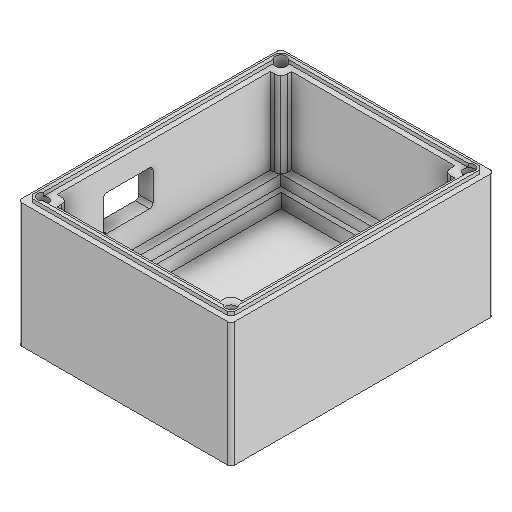
# Autodesk Inventor part: Box_bottom_v2
Saved by Autodesk Inventor 2026.1 (Build 301233020, 233B)
## iProperties
Created: 2025-09-17
Part Number: Box_bottom_v2
Material: Generic
Document SubType Name: Modeling
Designer: samuel
Density: 1 g/cm^3
Appearance: Default
Author: samuel
Autodesk Inventor part; units mm, degrees
ref_plane "YZ Plane" through (0, 0, 0) normal (1, 0, 0) x (0, 1, 0)
ref_plane "XZ Plane" through (0, 0, 0) normal (0, 1, 0) x (-1, 0, 0)
ref_plane "XY Plane" through (0, 0, 0) normal (0, 0, 1) x (1, 0, 0)
sketch "Sketch2" plane through (0, 0, 0) normal (0, 0, 1) x (1, 0, 0)
  line L0 (-30, -27) -> (30, -27)
  line L1 (30, -27) -> (30, 27)
  line L2 (30, 27) -> (-30, 27)
  line L3 (-30, 27) -> (-30, -27)
  line L4 (-30, -27) -> (30, 27) construction
  line L5 (30, -27) -> (-30, 27) construction
  line L6 (-30, 27) -> (30, 27)
  line L7 (30, 27) -> (30, 47)
  line L8 (30, 47) -> (-30, 47)
  line L9 (-30, 47) -> (-30, 27)
  line L10 (-25, -22) -> (25, -22)
  line L11 (25, -22) -> (25, 22)
  line L12 (25, 22) -> (-25, 22)
  line L13 (-25, 22) -> (-25, -22)
  point P0 (0, 0)
  dimension "d4" = 60
  dimension "d5" = 54
  dimension "d48" = 20
  dimension "d142" = 5
  constraints: 28 end point, 6 parallel, 3 perpendicular, 2 horizontal, 2 midpoint, 3 other
  measures "d4" distance of L2.end L1.end
  measures "d5" distance of L0.end L1.end
  measures "d48" distance of L7.end L6.end
  measures "d142" distance between parallel lines of L3 L13
extrude "Extrusion2" add sketch "Sketch2" along normal blind 35 contours L3 L2 L1 L0 | L9 L8 L7 L2 | L13 L12 L11 L10
shell "Shell1" thickness 4 removed faces 1 at (-10, 22.3333, 35)
sketch "Sketch11" plane through (-30, -27, 0) normal (-1, 0, 0) x (0, 0, 1)
  line L0 (28.5, 34) -> (18.5, 34)
  line L1 (18.5, 34) -> (18.5, 20)
  line L2 (18.5, 20) -> (28.5, 20)
  line L3 (28.5, 20) -> (28.5, 34)
  line L4 (28.5, 34) -> (18.5, 20) construction
  line L5 (18.5, 34) -> (28.5, 20) construction
  line L6 (0, 0) -> (35, 0) projected
  line L7 (0, 74) -> (0, 0) projected
  point P0 (0, 27)
  point P1 (23.5, 27)
  dimension "d65" = 10
  dimension "d66" = 14
  dimension "d67" = 20
  dimension "d68" = 18.5
  constraints: 12 end point, 2 midpoint, 2 parallel, 1 horizontal, 1 perpendicular
  measures "d65" distance of L2.end L1.end
  measures "d66" distance of L1.end L0.end
  measures "d67" distance between parallel lines of L6 L2
  measures "d68" distance between parallel lines of L7 L1
extrude "Extrusion9" cut sketch "Sketch11" against normal blind 5
sketch "Sketch12" plane through (-26, 43, 4) normal (0, 0, 1) x (1, 0, 0)
  line L0 (0, 0) -> (52, 0) projected
  line L1 (52, 0) -> (49, 0)
  line L2 (49, 0) -> (49, -3)
  line L3 (49, -3) -> (52, -3)
  line L4 (52, -3) -> (52, 0)
  line L5 (52, -66) -> (52, 0) projected
  line L6 (52, -66) -> (49, -66)
  line L7 (49, -66) -> (49, -63)
  line L8 (49, -63) -> (52, -63)
  line L9 (52, -63) -> (52, -66)
  point P0 (26, -43)
  point P1 (49, 0)
  dimension "d71" = 3
  dimension "d72" = 3
  dimension "d102" = 3
  dimension "d103" = 3
  constraints: 16 end point, 4 parallel, 2 horizontal, 2 perpendicular
  measures "d71" distance of L3.end L2.end
  measures "d72" distance of L2.end L1.end
  measures "d102" distance of L7.end L8.end
  measures "d103" distance of L6.end L7.end
extrude "Extrusion10" add sketch "Sketch12" along normal up to surface (31 mm away)
sketch "Sketch20" plane through (0, 0, 35) normal (0, 0, 1) x (1, 0, 0)
  circle A0 centre (-26.5, 43.5) radius 1.5 projected
  circle A1 centre (26.5, -23.5) radius 1.5 projected
  line L0 (-26.5, 43.5) -> (26.5, 43.5)
  line L1 (26.5, 43.5) -> (26.5, -23.5)
  line L2 (26.5, -23.5) -> (-26.5, -23.5)
  line L3 (-26.5, -23.5) -> (-26.5, 43.5)
  line L4 (27.5, 44.5) -> (-27.5, 44.5)
  line L5 (-27.5, 44.5) -> (-27.5, -24.5)
  line L6 (-27.5, -24.5) -> (27.5, -24.5)
  line L7 (27.5, -24.5) -> (27.5, 44.5)
  circle A2 centre (26.5, 43.5) radius 1.5
  circle A3 centre (-26.5, -23.5) radius 1.5
  line L8 (-28.5, 45.5) -> (28.5, 45.5)
  line L9 (28.5, 45.5) -> (28.5, -25.5)
  line L10 (28.5, -25.5) -> (-28.5, -25.5)
  line L11 (-28.5, -25.5) -> (-28.5, 45.5)
  point P0 (0, 0)
  point P1 (27.5, 42.382)
  point P2 (26.5, 42)
  point P3 (26.5, -22)
  point P4 (27.5, -22.382)
  point P5 (25, 43.5)
  point P6 (25.3819, 44.5)
  point P7 (-25.382, 44.5)
  point P8 (-25, 43.5)
  point P9 (-25, -23.5)
  point P10 (-25.382, -24.5)
  point P11 (25.3819, -24.5)
  point P12 (25, -23.5)
  point P13 (-27.5, -22.382)
  point P14 (-26.5, -22)
  point P15 (-26.5, 42)
  point P16 (-27.5, 42.382)
  dimension "d133" = 1
  dimension "d134" = 3
  dimension "d135" = 3
  dimension "d138" = 1
  constraints: 24 end point, 6 parallel, 3 perpendicular, 2 centre point, 2 coincident, 1 horizontal, 6 other
  measures "d133" distance between parallel lines of L0 L4
  measures "d134" diameter of A2
  measures "d135" diameter of A3
  measures "d138" distance between parallel lines of L4 L8
extrude "Extrusion13" add sketch "Sketch20" along normal blind 1
mirror "Mirror10" about plane through (0, 0, 0) normal (1, 0, 0) of "Extrusion10"
sketch "Sketch22" plane through (0, 0, 35) normal (0, 0, 1) x (1, 0, 0)
  arc A0 (-27.5, -22.382) -> (-25.382, -24.5) centre (-26.5, -23.5) ccw projected
  line L0 (-25.382, -24.5) -> (-28.5, -24.5)
  line L1 (-28.5, 45.5) -> (-28.5, -25.5) projected
  line L2 (-27.5, -22.382) -> (-27.5, 42.382) projected
  line L3 (-27.5, -22.382) -> (-27.5, -25.5)
  line L4 (-28.5, -25.5) -> (28.5, -25.5) projected
  circle A1 centre (-26.5, -23.5) radius 1.5
  line L5 (-25.382, 44.5) -> (25.3819, 44.5) projected
  line L6 (-25.165, 44.5) -> (-28.5, 44.5)
  line L7 (-27.5, 42.2455) -> (-27.5, 45.5)
  line L8 (-27.5, 44.5) -> (-25.5, 42.5)
  line L9 (-27.5, 44.5) -> (-24.6716, 44.5) construction
  circle A2 centre (-26.5, 43.5) radius 1.5
  arc A3 (-25.382, 44.5) -> (-27.5, 42.382) centre (-26.5, 43.5) ccw projected
  point P0 (0, 0)
  point P1 (-25.382, -24.5)
  dimension "d148" = 45
  dimension "d149" = 3
  dimension "d150" = 0
  constraints: 12 end point, 8 point on line, 2 horizontal, 2 perpendicular, 1 centre point, 1 coincident, 1 equal length, 1 midpoint, 3 other
  measures "d148" angle of L8 L9
  measures "d149" diameter of A2
  measures "d150" distance of A3.centre A2.centre
extrude "Extrusion16" cut sketch "Sketch22" against normal blind 10 contours L3 L0 A0 | A1 L0 L3 | L0 L3 A0 | L0 A0 L3 | A2 L6 L7 | L7 L6 A2 | L7 A2 L6 | L6 A2 L7
sketch "Sketch21" plane through (23, -20, 4) normal (0, 0, 1) x (1, 0, 0)
  line L0 (-48.9438, -3) -> (3.0062, -3)
  line L1 (3.0062, -3) -> (3.0062, 63)
  line L2 (3.0062, 63) -> (-48.9438, 63)
  line L3 (-48.9438, 63) -> (-48.9438, -3)
  line L4 (-46, -0.0562) -> (0.0624, -0.0562)
  line L5 (0.0624, -0.0562) -> (0.0624, 60.0562)
  line L6 (0.0624, 60.0562) -> (-46, 60.0562)
  line L7 (-46, 60.0562) -> (-46, -0.0562)
  line L8 (-43.5, 2.4438) -> (-2.4376, 2.4438)
  line L9 (-2.4376, 2.4438) -> (-2.4376, 57.5562)
  line L10 (-2.4376, 57.5562) -> (-43.5, 57.5562)
  line L11 (-43.5, 57.5562) -> (-43.5, 2.4438)
  point P0 (-23, 20)
  dimension "d145" = 2.5
  constraints: 24 end point, 6 parallel, 3 perpendicular, 1 horizontal, 6 other
  measures "d145" distance between parallel lines of L7 L11
extrude "Extrusion14" add sketch "Sketch21" along normal blind 7 contours L3 L2 L1 L0
extrude "Extrusion15" add sketch "Sketch21" along normal blind 4 contours L7 L6 L5 L4
fillet "Fillet11" radius 1 8 edges at (-30, 47, 17.5) (-30, -27, 17.5) (30, -27, 17.5) (30, 47, 17.5) (-28, 7, 28.5) (-28, 7, 18.5) (-28, -7, 18.5) (-28, -7, 28.5)
mirror "Mirror11" about plane through (0, 0, 0) normal (1, 0, 0) of "Extrusion16"
chamfer "Chamfer6" distance 1 angle 45 4 edges at (-28.5, -25.5, 35.5) (28.5, -25.5, 35.5) (28.5, 45.5, 35.5) (-28.5, 45.5, 35.5)
sketch "Sketch23" plane through (0, 0, 35) normal (0, 0, 1) x (1, 0, 0)
  line L0 (-23, -20) -> (-25.9438, -20) projected
  line L1 (-23, -20) -> (-26, -20)
  line L2 (-26, -20) -> (-26, -23)
  line L3 (-26, -23) -> (-23, -23)
  line L4 (-23, -23) -> (-23, -20)
  line L5 (-23, -20) -> (-23, 40) projected
  line L6 (-26, -23) -> (-23, -20)
  line L7 (-26, -20) -> (-23, -23)
  line L8 (-24.5, -21.5) -> (24.5, -21.5)
  line L9 (24.5, -21.5) -> (24.5, 41.5)
  line L10 (24.5, 41.5) -> (-24.5, 41.5)
  line L11 (-24.5, 41.5) -> (-24.5, -21.5)
  line L12 (23.5, 40.5) -> (23.5, -20.5)
  line L13 (23.5, -20.5) -> (-23.5, -20.5)
  line L14 (-23.5, -20.5) -> (-23.5, 40.5)
  line L15 (-23.5, 40.5) -> (23.5, 40.5)
  point P0 (0, 0)
  point P1 (-23.5, -20)
  point P2 (-23, -20.5)
  dimension "d156" = 3
  dimension "d157" = 49
  dimension "d158" = 63
  dimension "d164" = 1
  constraints: 28 end point, 6 parallel, 3 perpendicular, 2 horizontal, 1 midpoint, 3 other
  measures "d156" distance of L3.end L2.end
  measures "d157" distance of L10.end L9.end
  measures "d158" distance of L9.end L8.end
  measures "d164" distance between parallel lines of L9 L12
extrude "Extrusion17" cut sketch "Sketch23" against normal blind 27 contours L6 L14 L0 | L0 L14 L15 L12 L13 L4 | L4 L13 L6
fillet "Fillet12" radius 2 8 edges at (23, 40.5, 23) (23.5, 40, 23) (23, -20.5, 23) (23.5, -20, 23) (-23.5, 40, 23) (-23, 40.5, 23) (-23.5, -20, 23) (-23, -20.5, 23)
sketch "Sketch24" plane through (23, -20, 8) normal (0, 0, 1) x (1, 0, 0)
  line L0 (-43.5, 2.4438) -> (-43.5, 57.5562) projected
  line L1 (-2.4376, 57.5562) -> (-2.4376, 2.4438) projected
  line L2 (-43.5, 57.5562) -> (-2.4376, 57.5562)
  line L3 (-2.4376, 57.5562) -> (-2.4376, 2.4438)
  line L4 (-2.4376, 2.4438) -> (-43.5, 2.4438)
  line L5 (-43.5, 2.4438) -> (-43.5, 57.5562)
  line L6 (-0.9376, 59.0562) -> (-45, 59.0562)
  line L7 (-45, 59.0562) -> (-45, 0.9438)
  line L8 (-45, 0.9438) -> (-0.9376, 0.9438)
  line L9 (-0.9376, 0.9438) -> (-0.9376, 59.0562)
  point P0 (-23, 20)
  dimension "d166" = 1.5
  constraints: 16 end point, 4 parallel, 2 perpendicular, 1 horizontal, 3 other
  measures "d166" distance between parallel lines of L2 L6
extrude "Extrusion18" cut sketch "Sketch24" against normal blind 4
body "Solid2"
